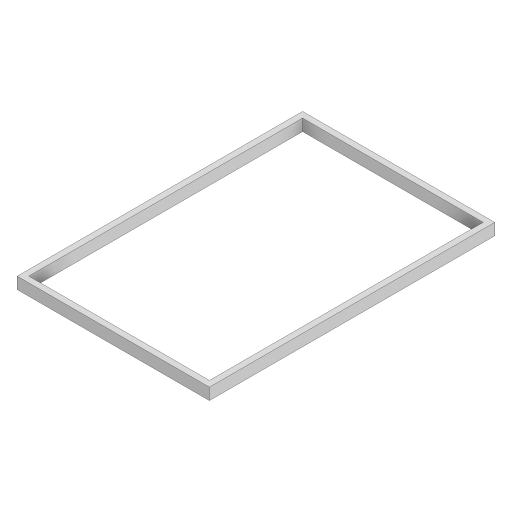
# Autodesk Inventor part: Base
Saved by Autodesk Inventor 2023 (Build 270158000, 158)
## iProperties
Created: 2022-09-15
Part Number: Base
Material: Generic
Document SubType Name: Modeling
Designer: Vking
Density: 1 g/cm^3
Appearance: Default
Author: Vking
Autodesk Inventor part; units mm, degrees
ref_plane "YZ Plane" through (0, 0, 0) normal (1, 0, 0) x (0, 1, 0)
ref_plane "XZ Plane" through (0, 0, 0) normal (0, 1, 0) x (-1, 0, 0)
ref_plane "XY Plane" through (0, 0, 0) normal (0, 0, 1) x (1, 0, 0)
sketch "Sketch1" plane through (0, 0, 0) normal (0, 1, 0) x (-1, 0, 0)
  line L0 (8.8462, 12.6468) -> (-30.5238, 12.6468)
  line L1 (-30.5238, 12.6468) -> (-30.5238, -47.0432)
  line L2 (-30.5238, -47.0432) -> (8.8462, -47.0432)
  line L3 (8.8462, -47.0432) -> (8.8462, 12.6468)
  line L4 (10.1162, 13.9168) -> (-31.7938, 13.9168)
  line L5 (-31.7938, 13.9168) -> (-31.7938, -48.3132)
  line L6 (-31.7938, -48.3132) -> (10.1162, -48.3132)
  line L7 (10.1162, -48.3132) -> (10.1162, 13.9168)
  point P0 (0, 0)
  dimension "d0" = 59.69
  dimension "d1" = 39.37
  dimension "d2" = 1.27
  constraints: 16 end point, 4 parallel, 2 perpendicular, 1 horizontal, 3 other
  measures "d0" distance of L2.end L0.start
  measures "d1" distance of L0.start L0.end
  measures "d2" distance between parallel lines of L3 L7
extrude "Extrusion1" add sketch "Sketch1" along normal blind 2.54
body "Solid1"
